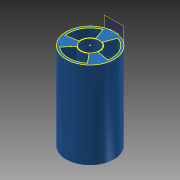
# Autodesk Inventor part: 知能ロボコンシリンダ
Saved by Autodesk Inventor 2013 (Build 170138000, 138)
## iProperties
Created: 2014-05-15
Part Number: 知能ロボコンシリンダ
Material: ABS プラスチック
Document SubType Name: Modeling
Designer: horumo136
Density: 1.06 g/cm^3
Mass: 61.8478 g
Surface Area: 517.048 cm^2
Volume: 58.347 cm^3
Author: horumo136
Autodesk Inventor part; units mm, degrees
ref_plane "YZ Plane" through (0, 0, 0) normal (1, 0, 0) x (0, 1, 0)
ref_plane "XZ Plane" through (0, 0, 0) normal (0, 1, 0) x (-1, 0, 0)
ref_plane "XY Plane" through (0, 0, 0) normal (0, 0, 1) x (1, 0, 0)
sketch "スケッチ1" plane through (0, 0, 0) normal (0, 0, 1) x (1, 0, 0)
  circle A0 centre (0, 0) radius 27.5
  dimension "d0" = 55
  constraints: 1 centre point, 1 coincident
  measures "d0" diameter of A0
extrude "押し出し1" add sketch "スケッチ1" along normal blind 100
sketch "スケッチ2" plane through (0, 0, 100) normal (0, 0, 1) x (1, 0, 0)
  circle A0 centre (0, 0) radius 27.5 projected
  circle A1 centre (0, 0) radius 25
  dimension "d3" = 50
  constraints: 1 centre point, 1 coincident
  measures "d3" diameter of A1
extrude "押し出し2" cut sketch "スケッチ2" against normal blind 97 contours A1
sketch "スケッチ3" plane through (0, 0, 3) normal (0, 0, 1) x (1, 0, 0)
  circle A0 centre (0, 0) radius 25 projected
  circle A1 centre (0, 0) radius 10.5
  circle A2 centre (0, 0) radius 11
  dimension "d6" = 21
  dimension "d7" = 22
  constraints: 2 centre point, 2 coincident
  measures "d6" diameter of A1
  measures "d7" diameter of A2
extrude "押し出し3" add sketch "スケッチ3" along normal blind 97 contours A2
sketch "スケッチ4" plane through (0, 0, 100) normal (0, 0, 1) x (1, 0, 0)
  circle A0 centre (0, 0) radius 25 projected
  circle A1 centre (0, 0) radius 27.5 projected
  circle A2 centre (0, 0) radius 11
  line L0 (0, 0) -> (0, 25)
  line L1 (0, 0) -> (8.5505, 23.4923)
  line L2 (0, 0) -> (25, 0) construction
  line L3 (0, 0) -> (-8.5505, 23.4923)
  line L4 (0, 0) -> (25, 0) construction
  line L5 (0, 0) -> (-21.6506, -12.5)
  line L6 (0, 0) -> (25, 0) construction
  line L7 (0, 0) -> (21.6506, -12.5)
  line L8 (0, 0) -> (25, 0) construction
  line L9 (0, 0) -> (-16.0697, -19.1511)
  line L10 (0, 0) -> (25, 0) construction
  line L11 (0, 0) -> (-24.6202, -4.3412)
  line L12 (0, 0) -> (25, 0) construction
  line L13 (0, 0) -> (24.6202, -4.3412)
  line L14 (0, 0) -> (25, 0) construction
  line L15 (0, 0) -> (16.0697, -19.1511)
  line L16 (0, 0) -> (25, 0) construction
  dimension "d10" = 22
  dimension "d11" = 70
  dimension "d12" = 110
  dimension "d13" = 150
  dimension "d14" = 30
  dimension "d15" = 130
  dimension "d16" = 170
  dimension "d17" = 10
  dimension "d18" = 50
  constraints: 34 end point, 8 equal length, 8 horizontal, 1 centre point, 1 coincident, 1 vertical, 10 other
  measures "d10" diameter of A2
  measures "d11" angle of L2 L1
  measures "d12" angle of L4 L3
  measures "d13" angle of L5 L6
  measures "d14" angle of L7 L8
  measures "d15" angle of L9 L10
  measures "d16" angle of L11 L12
  measures "d17" angle of L13 L14
  measures "d18" angle of L15 L16
extrude "押し出し4" add sketch "スケッチ4" against normal blind 15 contours L1 A2 L0 A0 | A0 L7 A2 L13 | L0 A2 L3 A0 | L1 L0 A2 | A0 L15 A2 L7 | A2 L7 L13 | L0 L3 A2 | L9 A2 L5 | L5 A2 L11 | L7 A2 L15 | L11 A2 L5 A0 | A2 L9 A0 L5
sketch "スケッチ5" plane through (0, 0, 100) normal (0, 0, 1) x (1, 0, 0)
  arc A0 (-6.7493, -8.0435) -> (6.7493, -8.0435) centre (0, 0) ccw projected
  line L0 (-6.7493, -8.0435) -> (0, 0) projected
  line L1 (0, 0) -> (-10.3405, -1.8233) projected
  arc A1 (-3.5912, 9.8668) -> (-10.3405, -1.8233) centre (0, 0) ccw projected
  line L2 (-3.5912, 9.8668) -> (0, 0) projected
  line L3 (0, 0) -> (3.5912, 9.8668) projected
  arc A2 (10.3405, -1.8233) -> (3.5912, 9.8668) centre (0, 0) ccw projected
  line L4 (10.3405, -1.8233) -> (0, 0) projected
  line L5 (0, 0) -> (6.7493, -8.0435) projected
  circle A3 centre (0, 0) radius 27.5 projected
  circle A4 centre (0, 0) radius 10.5
  constraints: 1 coincident, 3 other
extrude "押し出し5" cut sketch "スケッチ5" against normal blind 15 contours A4 L1 L0 | L5 L4 A4 | L2 A4 L3
sketch "スケッチ6" plane through (0, 0, 100) normal (0, 0, 1) x (1, 0, 0)
  circle A0 centre (0, 0) radius 27.5 projected
  line L0 (24.6202, -4.3412) -> (10.8329, -1.9101) projected
  arc A1 (10.8329, -1.9101) -> (3.7622, 10.3366) centre (0, 0) ccw projected
  line L1 (3.7622, 10.3366) -> (8.5505, 23.4923) projected
  arc A2 (24.6202, -4.3412) -> (8.5505, 23.4923) centre (0, 0) ccw projected
  arc A3 (-8.5505, 23.4923) -> (-24.6202, -4.3412) centre (0, 0) ccw projected
  line L2 (-8.5505, 23.4923) -> (-3.7622, 10.3366) projected
  arc A4 (-3.7622, 10.3366) -> (-10.8329, -1.9101) centre (0, 0) ccw projected
  line L3 (-10.8329, -1.9101) -> (-24.6202, -4.3412) projected
  arc A5 (-16.0697, -19.1511) -> (16.0697, -19.1511) centre (0, 0) ccw projected
  line L4 (-16.0697, -19.1511) -> (-7.0707, -8.4265) projected
  arc A6 (-7.0707, -8.4265) -> (7.0707, -8.4265) centre (0, 0) ccw projected
  line L5 (7.0707, -8.4265) -> (16.0697, -19.1511) projected
  circle A7 centre (0, 0) radius 10.5 projected
  point P0 (0, 27.5)
  constraints: 1 vertical alignment, 1 other
ref_plane "作業平面1" through (0, 27.5, 100) normal (0, 1, 0) x (-1, 0, 0)
sketch "スケッチ8" plane through (0, 27.5, 100) normal (0, 1, 0) x (-1, 0, 0)
  line L0 (-4.8637, 0) -> (5.1363, 0)
  line L1 (5.1363, 0) -> (5.1363, -70)
  line L2 (5.1363, -70) -> (-4.8637, -70)
  line L3 (-4.8637, -70) -> (-4.8637, 0)
  line L4 (27.5, 0) -> (-27.5, 0) projected
  line L5 (0, 0) -> (0, -6)
  line L6 (0.1363, -70) -> (0.1363, -64)
  point P0 (0, -100)
  dimension "d27" = 10
  dimension "d28" = 70
  dimension "d29" = 0
  dimension "d30" = 6
  dimension "d31" = 6
  constraints: 12 end point, 3 parallel, 2 coincident, 2 midpoint, 2 perpendicular, 1 horizontal
  measures "d27" distance of L1.end L2.end
  measures "d28" distance of L0.end L1.end
  measures "d29" distance between parallel lines of L0 L4
  measures "d30" distance of L5.start L5.end
  measures "d31" distance of L6.start L6.end
extrude "押し出し6" add sketch "スケッチ8" against normal blind 1
sketch "スケッチ9" plane through (0, 27.5, 100) normal (0, 1, 0) x (1, 0, 0)
  line L0 (4.8637, 0) -> (-5.1363, 0) projected
  line L1 (-5.1363, 0) -> (-5.1363, 70) projected
  line L2 (0, 70) -> (0, 65.5)
  line L3 (-0.1363, 0) -> (-0.1363, 4.5)
  point P0 (0, 100)
  dimension "d34" = 4.5
  dimension "d35" = 4.5
  constraints: 4 end point, 2 coincident, 2 parallel, 1 midpoint
  measures "d34" distance of L2.start L2.end
  measures "d35" distance of L3.start L3.end
hole "穴1" at (0, 27.5, 34.5) at (-0.1363, 27.5, 95.5) direction (0, -1, 0) diameter 3 depth 8 tip angle 118
thread "ねじ1" size "M3x0.5" class "6H" standard "ANSI Metric M Profile" full length
thread "ねじ2" size "M3x0.5" class "6H" standard "ANSI Metric M Profile" full length
sketch "スケッチ10" plane through (0, 27.5, 100) normal (0, 1, 0) x (1, 0, 0)
  circle A0 centre (0, 65.5) radius 1.5 projected
  circle A1 centre (-0.1363, 4.5) radius 1.5 projected
  line L0 (4.8637, 0) -> (-5.1363, 0) projected
  line L1 (4.8637, 70) -> (4.8637, 0) projected
  line L2 (0, 70) -> (4.8637, 70) projected
  line L3 (-5.1363, 70) -> (0, 70) projected
  line L4 (-5.1363, 0) -> (-5.1363, 70) projected
  point P0 (0, 100)
